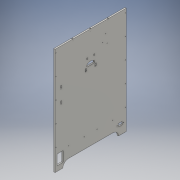
# Autodesk Inventor part: Bagsiden mk2
Saved by Autodesk Inventor 2016 (Build 200138000, 138)
## iProperties
Created: 2015-10-17
Part Number: Bagsiden mk2
Material: Generic
Document SubType Name: Modeling
Designer: iLyngklip
Density: 1 g/cm^3
Appearance: White
Author: iLyngklip
Autodesk Inventor part; units mm, degrees
ref_plane "YZ Plane" through (0, 0, 0) normal (1, 0, 0) x (0, 1, 0)
ref_plane "XZ Plane" through (0, 0, 0) normal (0, 1, 0) x (-1, 0, 0)
ref_plane "XY Plane" through (0, 0, 0) normal (0, 0, 1) x (1, 0, 0)
sketch "Sketch1" plane through (0, 0, 0) normal (1, 0, 0) x (0, 1, 0)
  line L0 (-160, 240) -> (160, 240)
  line L1 (160, 240) -> (160, -240)
  line L2 (160, -240) -> (-160, -240)
  line L3 (-160, -240) -> (-160, 240)
  point P0 (0, 0)
  dimension "d0" = 320
  dimension "d1" = 480
  dimension "d2" = 240
  dimension "d3" = 160
  constraints: 8 end point, 2 parallel, 1 horizontal, 1 perpendicular
  measures "d0" distance of L1.end L2.end
  measures "d1" distance of L0.end L1.end
  measures "d2" distance from line of point (0, 0) L2
  measures "d3" distance from line of point (0, 0) L1
extrude "6mm tykkelse" add sketch "Sketch1" along normal blind 6
sketch "Sketch2" plane through (6, 0, 0) normal (1, 0, 0) x (0, 0, -1)
  line L0 (-240, 160) -> (-240, -160) construction
  line L1 (-240, -160) -> (240, -160) construction
  line L2 (240, -160) -> (240, 160) construction
  line L3 (240, 160) -> (-240, 160) construction
  arc A0 (215, -100) -> (240, -125) centre (240, -100) ccw
  arc A1 (240, 125) -> (215, 100) centre (240, 100) ccw
  line L4 (215, 100) -> (215, -100)
  line L5 (240, 125) -> (240, -125)
  point P0 (0, 0)
  dimension "d6" = 50
  dimension "d7" = 50
  dimension "d8" = 60
  dimension "d9" = 60
  constraints: 4 end point, 4 point on circle, 4 point on line, 2 centre point, 1 collinear, 1 tangent, 1 vertical
  measures "d6" diameter of A1
  measures "d7" diameter of A0
  measures "d8" distance of L2.end A1.centre
  measures "d9" distance of L1.end A0.centre
extrude "Fødder" cut sketch "Sketch2" against normal up to surface (6 mm away)
sketch "Sketch3" plane through (6, 0, 0) normal (1, 0, 0) x (0, 0, -1)
  circle A0 centre (-224, -156) radius 1.5
  circle A1 centre (-132, -156) radius 1.5
  circle A2 centre (-40, -156) radius 1.5
  circle A3 centre (144, 156) radius 1.5
  circle A4 centre (52, 156) radius 1.5
  circle A5 centre (-40, 156) radius 1.5
  circle A6 centre (-132, 156) radius 1.5
  circle A7 centre (144, -156) radius 1.5
  line L0 (-169.5485, -156) -> (381.2467, -156) construction
  line L1 (-240, -160) -> (240, -160) projected
  line L2 (-156.9318, 156) -> (328.4718, 156) construction
  line L3 (240, 160) -> (-240, 160) projected
  line L4 (240, -160) -> (240, -125) projected
  circle A8 centre (52, -156) radius 1.5
  circle A9 centre (-224, 156) radius 1.5
  line L5 (240, 125) -> (240, 160) projected
  point P0 (0, 0)
  dimension "d12" = 4
  dimension "d13" = 3
  dimension "d14" = 3
  dimension "d15" = 3
  dimension "d16" = 3
  dimension "d17" = 3
  dimension "d18" = 3
  dimension "d19" = 3
  dimension "d20" = 3
  dimension "d21" = 4
  dimension "d22" = 96
  dimension "d26" = 3
  dimension "d28" = 3
  dimension "d29" = 96
  dimension "d226" = 92
  dimension "d227" = 92
  dimension "d228" = 92
  dimension "d229" = 92
  dimension "d230" = 92
  dimension "d231" = 92
  dimension "d232" = 92
  dimension "d233" = 92
  constraints: 10 centre point, 10 point on line, 4 end point, 2 horizontal
  measures "d12" distance between parallel lines of L1 L0
  measures "d13" diameter of A7
  measures "d14" diameter of A2
  measures "d15" diameter of A1
  measures "d16" diameter of A0
  measures "d17" diameter of A3
  measures "d18" diameter of A4
  measures "d19" diameter of A5
  measures "d20" diameter of A6
  measures "d21" distance between parallel lines of L3 L2
  measures "d22" distance from line of L4 A7.centre
  measures "d26" diameter of A8
  measures "d28" diameter of A9
  measures "d29" distance from line of L5 A3.centre
  measures "d226" distance of A8.centre A7.centre
  measures "d227" distance of A8.centre A2.centre
  measures "d228" distance of A2.centre A1.centre
  measures "d229" distance of A1.centre A0.centre
  measures "d230" distance of A4.centre A3.centre
  measures "d231" distance of A5.centre A4.centre
  measures "d232" distance of A6.centre A5.centre
  measures "d233" distance of A9.centre A6.centre
extrude "Monteringshuller" cut sketch "Sketch3" against normal up to surface (6 mm away)
sketch "Sketch5" plane through (0, 0, 0) normal (-1, 0, 0) x (0, 0, 1)
  circle A0 centre (218, 142) radius 4 construction
  circle A1 centre (218, -136) radius 4 construction
  line L0 (240, -160) -> (240, 160) projected
  line L1 (-240, -160) -> (240, -160) projected
  line L2 (240, 160) -> (-240, 160) projected
  circle A2 centre (218, -136) radius 8
  circle A3 centre (218, 142) radius 8
  point P0 (0, 0)
  dimension "d43" = 8
  dimension "d52" = 22
  dimension "d53" = 24
  dimension "d54" = 22
  dimension "d55" = 18
  dimension "d82" = 16
  dimension "d83" = 16
  constraints: 4 centre point, 2 coincident
  measures "d43" diameter of A0
  measures "d52" distance from line of L0 A1.centre
  measures "d53" distance from line of L1 A1.centre
  measures "d54" distance from line of L0 A0.centre
  measures "d55" distance from line of L2 A0.centre
  measures "d82" diameter of A2
  measures "d83" diameter of A3
sketch "Sketch6" plane through (6, 0, 0) normal (1, 0, 0) x (0, 0, -1)
  circle A0 centre (-19, -133) radius 2.5 construction
  circle A1 centre (-79, -133) radius 2.5 construction
  line L0 (-99.3485, -133) -> (-215.3198, -133) construction
  arc A2 (-84, -130.5) -> (-84, -135.5) centre (-84, -133) ccw
  arc A3 (-74, -135.5) -> (-74, -130.5) centre (-74, -133) ccw
  arc A4 (-24, -130.5) -> (-24, -135.5) centre (-24, -133) ccw
  arc A5 (-14, -135.5) -> (-14, -130.5) centre (-14, -133) ccw
  line L1 (-240, -160) -> (240, -160) projected
  line L2 (-240, 160) -> (-240, -160) projected
  line L3 (-84, -130.5) -> (-74, -130.5)
  line L4 (-84, -135.5) -> (-74, -135.5)
  line L5 (-24, -130.5) -> (-14, -130.5)
  line L6 (-24, -135.5) -> (-14, -135.5)
  point P0 (0, 0)
  dimension "d60" = 5
  dimension "d61" = 5
  dimension "d62" = 5
  dimension "d63" = 5
  dimension "d64" = 5
  dimension "d65" = 5
  dimension "d66" = 60
  dimension "d67" = 27
  dimension "d68" = 161
  dimension "d69" = 5
  dimension "d70" = 10
  dimension "d71" = 5
  dimension "d72" = 10
  constraints: 10 end point, 8 point on circle, 8 tangent, 6 centre point, 6 point on line, 1 horizontal
  measures "d60" diameter of A1
  measures "d61" diameter of A2
  measures "d62" diameter of A3
  measures "d63" diameter of A0
  measures "d64" diameter of A5
  measures "d65" diameter of A4
  measures "d66" distance of A1.centre A0.centre
  measures "d67" distance between parallel lines of L1 L0
  measures "d68" distance from line of L2 A1.centre
  measures "d69" distance of A1.centre A3.centre
  measures "d70" distance of A3.centre A2.centre
  measures "d71" distance of A0.centre A4.centre
  measures "d72" distance of A4.centre A5.centre
extrude "Motor montage" cut sketch "Sketch6" against normal blind 10
sketch "Sketch7" plane through (6, 0, 0) normal (1, 0, 0) x (0, 0, -1)
  circle A0 centre (-131, -15.75) radius 1.65 construction
  circle A1 centre (-131, 15.75) radius 1.65 construction
  line L0 (-131, 15.75) -> (-131, -15.75) construction
  line L1 (240, 160) -> (-240, 160) projected
  line L2 (-240, 160) -> (-240, -160) projected
  arc A2 (-133.5, 17.4) -> (-133.5, 14.1) centre (-133.5, 15.75) ccw
  arc A3 (-128.5, 14.1) -> (-128.5, 17.4) centre (-128.5, 15.75) ccw
  arc A4 (-128.5, -17.4) -> (-128.5, -14.1) centre (-128.5, -15.75) ccw
  arc A5 (-133.5, -14.1) -> (-133.5, -17.4) centre (-133.5, -15.75) ccw
  line L3 (-133.5, -14.1) -> (-128.5, -14.1)
  line L4 (-133.5, -17.4) -> (-128.5, -17.4)
  line L5 (-133.5, 14.1) -> (-128.5, 14.1)
  line L6 (-133.5, 17.4) -> (-128.5, 17.4)
  point P0 (0, 0)
  dimension "d75" = 31.5
  dimension "d76" = 3.3
  dimension "d77" = 3.3
  dimension "d78" = 144.25
  dimension "d79" = 109
  dimension "d121" = 3.3
  dimension "d122" = 3.3
  dimension "d123" = 2.5
  dimension "d124" = 2.5
  dimension "d125" = 5
  dimension "d126" = 3.3
  dimension "d127" = 3.3
  constraints: 10 end point, 8 point on circle, 8 tangent, 6 centre point, 4 horizontal alignment, 2 vertical alignment, 1 vertical
  measures "d75" distance of L0.end L0.start
  measures "d76" diameter of A1
  measures "d77" diameter of A0
  measures "d78" distance from line of L1 L0.start
  measures "d79" distance from line of L2 L0.start
  measures "d121" diameter of A5
  measures "d122" diameter of A2
  measures "d123" distance of A5.centre L0.end
  measures "d124" distance of A4.centre L0.end
  measures "d125" distance of A5.centre A4.centre
  measures "d126" diameter of A4
  measures "d127" diameter of A3
extrude "Z-Gevind holder montage hul" cut sketch "Sketch7" against normal blind 10
extrude "Leje huller" cut sketch "Sketch5" against normal blind 3.5
sketch "Sketch8" plane through (0, 0, 0) normal (-1, 0, 0) x (0, 0, 1)
  arc A0 (230.8, 82.75) -> (229.302, 81.3277) centre (230.8, 81.25) ccw
  arc A1 (233.679, 81.5) -> (232.2, 82.75) centre (232.2, 81.25) ccw
  line L0 (230.8, 82.75) -> (232.2, 82.75)
  line L1 (232.2, 77.25) -> (230.8, 77.25)
  arc A2 (229.302, 78.6723) -> (230.8, 77.25) centre (230.8, 78.75) ccw
  arc A3 (229.302, 81.3277) -> (229.302, 78.6723) centre (230, 80) ccw
  arc A4 (232.2, 77.25) -> (233.679, 78.5) centre (232.2, 78.75) ccw
  line L2 (240, 78.5) -> (233.679, 78.5)
  line L3 (230, 80) -> (240, 80) construction
  line L4 (240, 81.5) -> (233.679, 81.5)
  arc A5 (230.8, -77.25) -> (229.302, -78.6723) centre (230.8, -78.75) ccw
  arc A6 (233.679, -78.5) -> (232.2, -77.25) centre (232.2, -78.75) ccw
  line L5 (230.8, -77.25) -> (232.2, -77.25)
  line L6 (232.2, -82.75) -> (230.8, -82.75)
  arc A7 (229.302, -81.3277) -> (230.8, -82.75) centre (230.8, -81.25) ccw
  arc A8 (229.302, -78.6723) -> (229.302, -81.3277) centre (230, -80) ccw
  arc A9 (232.2, -82.75) -> (233.679, -81.5) centre (232.2, -81.25) ccw
  line L7 (240, -81.5) -> (233.679, -81.5)
  line L8 (230, -80) -> (240, -80) construction
  line L9 (240, -78.5) -> (233.679, -78.5)
  arc A10 (230.8, 2.75) -> (229.302, 1.3277) centre (230.8, 1.25) ccw
  arc A11 (233.679, 1.5) -> (232.2, 2.75) centre (232.2, 1.25) ccw
  line L10 (230.8, 2.75) -> (232.2, 2.75)
  line L11 (232.2, -2.75) -> (230.8, -2.75)
  arc A12 (229.302, -1.3277) -> (230.8, -2.75) centre (230.8, -1.25) ccw
  arc A13 (229.302, 1.3277) -> (229.302, -1.3277) centre (230, 0) ccw
  arc A14 (232.2, -2.75) -> (233.679, -1.5) centre (232.2, -1.25) ccw
  line L12 (240, -1.5) -> (233.679, -1.5)
  line L13 (230, 0) -> (240, 0) construction
  line L14 (240, 1.5) -> (233.679, 1.5)
  line L15 (240, 160) -> (-240, 160) projected
  line L16 (240, 78.5) -> (240, 81.5)
  line L17 (240, 160) -> (240, -160) projected
  line L18 (240, 1.5) -> (240, -1.5)
  line L19 (240, -78.5) -> (240, -81.5)
  point P0 (0, 0)
  dimension "d128" = 80
  dimension "d129" = 160
  dimension "d130" = 240
  constraints: 36 end point, 30 point on circle, 15 centre point, 3 collinear
  measures "d128" distance between parallel lines of L15 L3
  measures "d129" distance between parallel lines of L15 L13
  measures "d130" distance between parallel lines of L15 L8
extrude "Låg montage huller" cut sketch "Sketch8" against normal blind 5
sketch "Sketch10" plane through (6, 0, 0) normal (1, 0, 0) x (0, 0, -1)
  circle A0 centre (-146.2747, 74.5256) radius 1.5 projected
  circle A1 centre (-159.2715, 53.782) radius 1.5 projected
  circle A2 centre (-187.2483, 67.5978) radius 1.5 projected
  point P0 (0, 0)
extrude "Extruder-mount" cut sketch "Sketch10" against normal up to surface (6 mm away)
sketch "Sketch11" plane through (6, 0, 0) normal (1, 0, 0) x (0, 0, -1)
  line L0 (-240, -160) -> (240, -160) projected
  line L1 (240, 160) -> (-240, 160) projected
  line L2 (240, 125) -> (240, 160) projected
  arc A0 (-108.881, 16.0739) -> (-108.881, -16.0739) centre (-90, 0) ccw
  line L3 (-107.8695, -16.5959) -> (-100.9272, -17.2033)
  arc A1 (-108.881, -16.0739) -> (-107.8695, -16.5959) centre (-107.7388, -15.1016) ccw
  arc A2 (-100.9272, -17.2033) -> (-99.2964, -15.709) centre (-100.7964, -15.709) ccw
  line L4 (-99.2964, -15.709) -> (-99.2964, 15.709)
  line L5 (-100.9272, 17.2033) -> (-107.8695, 16.5959)
  arc A3 (-107.8695, 16.5959) -> (-108.881, 16.0739) centre (-107.7388, 15.1016) ccw
  arc A4 (-99.2964, 15.709) -> (-100.9272, 17.2033) centre (-100.7964, 15.709) ccw
  line L6 (-95.5, -20.4081) -> (-95.5, -23.4578)
  arc A5 (-93.7115, -18.9361) -> (-95.5, -20.4081) centre (-94, -20.4081) ccw
  arc A6 (-93.7115, -18.9361) -> (-84.8967, -18.6094) centre (-90, 0) ccw
  arc A7 (-83, -20.0559) -> (-84.8967, -18.6094) centre (-84.5, -20.0559) ccw
  line L7 (-83, -23.1521) -> (-83, -20.0559)
  arc A8 (-84.1533, -24.6115) -> (-83, -23.1521) centre (-84.5, -23.1521) ccw
  arc A9 (-94.2521, -24.9365) -> (-84.1533, -24.6115) centre (-90, 0) ccw
  arc A10 (-95.5, -23.4578) -> (-94.2521, -24.9365) centre (-94, -23.4578) ccw
  line L8 (-83, 20.0559) -> (-83, 23.1521)
  arc A11 (-84.8967, 18.6094) -> (-83, 20.0559) centre (-84.5, 20.0559) ccw
  arc A12 (-84.8967, 18.6094) -> (-93.7115, 18.9361) centre (-90, 0) ccw
  arc A13 (-95.5, 20.4081) -> (-93.7115, 18.9361) centre (-94, 20.4081) ccw
  line L9 (-95.5, 23.4578) -> (-95.5, 20.4081)
  arc A14 (-94.2521, 24.9365) -> (-95.5, 23.4578) centre (-94, 23.4578) ccw
  arc A15 (-84.1533, 24.6115) -> (-94.2521, 24.9365) centre (-90, 0) ccw
  arc A16 (-83, 23.1521) -> (-84.1533, 24.6115) centre (-84.5, 23.1521) ccw
  point P0 (0, 0)
  point P1 (-83.6888, -5.5936)
  dimension "d6" = 50
  dimension "d7" = 50
  dimension "d8" = 60
  dimension "d9" = 60
  dimension "d147" = 320
  dimension "d169" = 1.5
  dimension "d170" = 24.7964
  dimension "d171" = 1.5
  dimension "d172" = 1.5
  dimension "d173" = 1.5
  dimension "d174" = 31.4179
  dimension "d175" = 85
  dimension "d176" = 30.2032
  dimension "d177" = 6.9424
  dimension "d178" = 1.5
  dimension "d179" = 1.5
  dimension "d180" = 92.123
  dimension "d181" = 1.5
  dimension "d182" = 19.2964
  dimension "d183" = 25.2964
  dimension "d184" = 1.5
  dimension "d185" = 3.0962
  dimension "d186" = 9.5
  dimension "d187" = 88.157
  dimension "d188" = 1.5
  dimension "d189" = 25.2964
  dimension "d190" = 19.2964
  dimension "d191" = 12.5
  dimension "d192" = 1.1533
  dimension "d193" = 12.5
  dimension "d194" = 12.5
  dimension "d195" = 85
  dimension "d196" = 9.2964
  dimension "d197" = 160
  dimension "d198" = 330
  dimension "d199" = 0.6888
  dimension "d200" = 0.6888
  constraints: 34 point on circle, 24 tangent, 17 centre point, 14 end point, 3 equal radius, 2 coincident, 2 parallel, 1 concentric
  measures "d147" distance between parallel lines of L0 L1
  measures "d169" radius of A1
  measures "d170" radius of A0
  measures "d171" radius of A3
  measures "d172" radius of A4
  measures "d173" radius of A2
  measures "d174" distance of A4.centre A2.centre
  measures "d175" angle of L5 L4
  measures "d176" distance of A1.centre A3.centre
  measures "d177" horizontal distance of A1.centre A2.centre
  measures "d178" radius of A5
  measures "d179" radius of A10
  measures "d181" radius of A7
  measures "d182" radius of A6
  measures "d183" radius of A9
  measures "d184" radius of A8
  measures "d185" distance of A7.centre A8.centre
  measures "d186" horizontal distance of A10.centre A8.centre
  measures "d188" radius of A16
  measures "d189" radius of A15
  measures "d190" radius of A12
  measures "d191" distance between parallel lines of L9 L8
  measures "d192" distance from line of A15.start L8
  measures "d193" distance from line of L7.end L6
  measures "d194" distance from line of L7.start L6
  measures "d195" angle of L4 L3
  measures "d196" distance from line of A0.centre L4
  measures "d197" distance from line of L1 A0.centre
  measures "d198" distance from line of L2 A0.centre
  measures "d199" distance from line of point (-83.689, -5.594) L8
  measures "d200" distance from line of point (-83.689, -5.594) L7
extrude "Filament holder mount" cut sketch "Sketch11" against normal up to surface (6 mm away)
sketch "Sketch12" plane through (0, 0, 0) normal (-1, 0, 0) x (0, 0, 1)
  line L0 (-166, 107.2792) -> (-166, -112.2374) construction
  line L1 (-240, 160) -> (-240, 125) projected
  circle A0 centre (-166, 99) radius 1.5
  line L2 (-166, 0) -> (-152.3363, 0) construction
  circle A1 centre (-166, 29) radius 1.5
  circle A2 centre (-166, -29) radius 1.5
  circle A3 centre (-166, -99) radius 1.5
  point P0 (0, 0)
  dimension "d203" = 74
  dimension "d204" = 3
  dimension "d205" = 61
  dimension "d206" = 70
  dimension "d207" = 29
  dimension "d208" = 29
  dimension "d209" = 70
  constraints: 5 point on line, 4 centre point, 4 end point, 3 equal radius, 1 horizontal, 1 parallel, 1 vertical
  measures "d203" distance between parallel lines of L1 L0
  measures "d204" diameter of A0
  measures "d205" vertical distance of L1.start A0.centre
  measures "d206" distance of A0.centre A1.centre
  measures "d207" distance from line of L2 A1.centre
  measures "d208" distance from line of A2.centre L2
  measures "d209" distance of A3.centre A2.centre
extrude "Midterplade monteringshuller" cut sketch "Sketch12" against normal blind 10
sketch "Sketch13" plane through (6, 0, 0) normal (1, 0, 0) x (0, 0, -1)
  line L0 (178.5, -150.8) -> (178.1, -150.8)
  line L1 (173.3, -150.8) -> (178.1, -150.8)
  arc A0 (172.1, -149.6) -> (173.3, -150.8) centre (173.3, -149.6) ccw
  line L2 (172.1, -144.8) -> (172.1, -149.6)
  line L3 (178.1, -123.6) -> (178.5, -123.6)
  line L4 (172.1, -124.8) -> (172.1, -129.6)
  arc A1 (173.3, -123.6) -> (172.1, -124.8) centre (173.3, -124.8) ccw
  line L5 (178.1, -123.6) -> (173.3, -123.6)
  line L6 (204.4, -150.8) -> (186, -150.8)
  line L7 (186, -123.6) -> (204.4, -123.6)
  line L8 (172.1, -144.8) -> (172.1, -129.6)
  line L9 (214.2, -123.6) -> (215.4, -123.6)
  arc A2 (217.9, -126.1) -> (215.4, -123.6) centre (215.4, -126.1) ccw
  line L10 (217.9, -126.1) -> (217.9, -148.3)
  arc A3 (215.4, -150.8) -> (217.9, -148.3) centre (215.4, -148.3) ccw
  line L11 (215.4, -150.8) -> (214.2, -150.8)
  line L12 (214.2, -123.6) -> (204.4, -123.6)
  line L13 (186, -123.6) -> (178.5, -123.6)
  line L14 (178.5, -150.8) -> (186, -150.8)
  line L15 (204.4, -150.8) -> (214.2, -150.8)
  point P0 (0, 0)
  constraints: 32 end point, 9 horizontal, 8 point on circle, 4 centre point, 4 vertical, 2 collinear, 1 parallel, 28 other
extrude "Strøm-tilslutning" cut sketch "Sketch13" against normal up to surface (6 mm away)
sketch "USB Sketch" plane through (0, 0, 0) normal (-1, 0, 0) x (0, 0, 1)
  line L0 (-205, 147) -> (-205, 119)
  line L1 (-191, 119) -> (-191, 147)
  arc A0 (-203, 119) -> (-193, 119) centre (-198, 119) ccw
  arc A1 (-193, 147) -> (-203, 147) centre (-198, 147) ccw
  line L2 (-191, 147) -> (-193, 147)
  line L3 (-203, 147) -> (-205, 147)
  line L4 (-205, 119) -> (-203, 119)
  line L5 (-193, 119) -> (-191, 119)
  line L6 (-191, 141.5) -> (-205, 141.5)
  line L7 (-205, 141.5) -> (-205, 124.5)
  line L8 (-205, 124.5) -> (-191, 124.5)
  line L9 (-191, 124.5) -> (-191, 141.5)
  line L10 (-240, 160) -> (-240, 125) projected
  line L11 (240, 160) -> (-240, 160) projected
  line L12 (-179.0585, 152) -> (-231.6448, 152) construction
  circle A2 centre (-198, 147) radius 1.5
  circle A3 centre (-198, 119) radius 1.5
  point P0 (0, 0)
  point P1 (-192, 119)
  point P2 (-204, 119)
  point P3 (-204, 147)
  point P4 (-192, 147)
  dimension "d252" = 28
  dimension "d253" = 14
  dimension "d254" = 17
  dimension "d255" = 10.5
  dimension "d256" = 10.5
  dimension "d258" = 2
  dimension "d264" = 35
  dimension "d266" = 8
  dimension "d267" = 3
  dimension "d268" = 3
  constraints: 22 end point, 7 parallel, 4 centre point, 4 horizontal, 4 horizontal alignment, 4 midpoint, 4 point on circle, 3 perpendicular, 2 coincident, 2 equal length, 2 point on line, 1 equal radius, 1 tangent, 1 vertical alignment
  measures "d252" distance of A0.centre A1.centre
  measures "d253" distance between parallel lines of L0 L1
  measures "d254" distance between parallel lines of L6 L8
  measures "d258" distance of L1.end L2.end
  measures "d264" distance between parallel lines of L10 L7
  measures "d266" distance between parallel lines of L11 L12
  measures "d267" diameter of A2
  measures "d268" diameter of A3
extrude "USB Undersænkning" cut sketch "USB Sketch" against normal blind 5 contours L3 A1 L2 L1 L6 L0 | L6 L1 L8 L0 | L8 L1 L5 A0 L4 L0 | A2 | A3
extrude "Extrusion17" cut sketch "USB Sketch" against normal up to surface (6 mm away) contours L6 L1 L8 L0 | A2 | A3
fillet "Fillet2" radius 1.5 8 edges at (2.5, 119, -191) (5.5, 124.5, -191) (5.5, 141.5, -191) (2.5, 147, -191) (2.5, 147, -205) (2.5, 119, -205) (5.5, 124.5, -205) (5.5, 141.5, -205)
equation "\"d2\" = 0.5 * d1"
equation "\"d3\" = 0.5 * d0"
equation "\"d6\" = d7"
equation "\"d9\" = d8"
equation "\"d14\" = d13"
equation "\"d15\" = d13"
equation "\"d16\" = d13"
equation "\"d17\" = d13"
equation "\"d18\" = d13"
equation "\"d19\" = d13"
equation "\"d20\" = d13"
equation "\"d21\" = d12"
equation "\"d26\" = d13"
equation "\"d28\" = d13"
equation "\"d29\" = d22"
equation "\"d61\" = d60"
equation "\"d62\" = d60"
equation "\"d64\" = d63"
equation "\"d65\" = d64"
equation "\"d70\" = 2 * d69"
equation "\"d71\" = d69"
equation "\"d72\" = 2 * d65"
equation "\"d76\" = d77"
equation "\"d121\" = d77"
equation "\"d122\" = d77"
equation "\"d123\" = d124"
equation "\"d126\" = d77"
equation "\"d127\" = d77"
equation "\"d54\" = d52"
body "Solid1"
